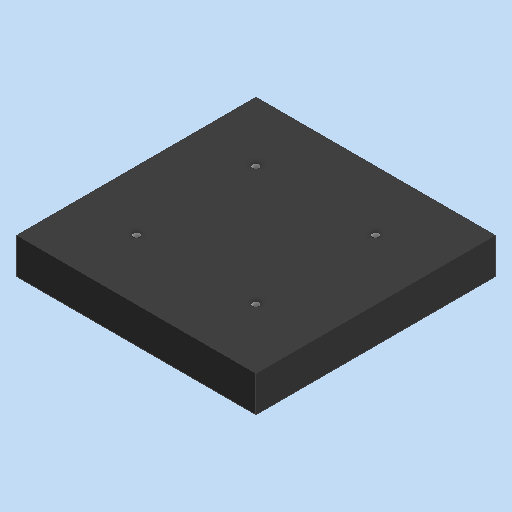
# Autodesk Inventor part: 底座
Saved by Autodesk Inventor 2026.2 (Build 302298010, 298A)
## iProperties
Created: 2026-03-16
Part Number: 底座
Material: 常规
Document SubType Name: Modeling
Designer: liu
Density: 1 g/cm^3
Appearance: 默认
Author: liu
Autodesk Inventor part; units mm, degrees
ref_plane "YZ Plane" through (0, 0, 0) normal (1, 0, 0) x (0, 1, 0)
ref_plane "XZ Plane" through (0, 0, 0) normal (0, 1, 0) x (-1, 0, 0)
ref_plane "XY Plane" through (0, 0, 0) normal (0, 0, 1) x (1, 0, 0)
sketch "草图1" plane through (0, 0, 0) normal (0, 1, 0) x (-1, 0, 0)
  line L0 (42.1224, 59.3469) -> (-57.8776, 59.3469)
  line L1 (-57.8776, 59.3469) -> (-57.8776, -40.6531)
  line L2 (-57.8776, -40.6531) -> (42.1224, -40.6531)
  line L3 (42.1224, -40.6531) -> (42.1224, 59.3469)
  point P0 (0, 0)
  dimension "d0" = 100
  dimension "d1" = 100
  constraints: 8 end point, 2 parallel, 1 horizontal, 1 perpendicular
  measures "d0" distance of L2.end L0.start
  measures "d1" distance of L1.end L2.end
extrude "拉伸1" add sketch "草图1" along normal blind 15
sketch "草图2" plane through (0, 15, 0) normal (0, 1, 0) x (1, 0, 0)
  circle A0 centre (-17.1224, -34.3469) radius 1.5
  line L0 (-42.1224, 40.6531) -> (-42.1224, -59.3469) projected
  line L1 (-42.1224, -59.3469) -> (57.8776, -59.3469) projected
  circle A1 centre (32.8776, -34.3469) radius 1.5
  circle A2 centre (32.8776, 15.6531) radius 1.5
  circle A3 centre (-17.1224, 15.6531) radius 1.5
  point P0 (0, 0)
  dimension "d4" = 3
  dimension "d5" = 25
  dimension "d6" = 25
  dimension "d9" = 50
  dimension "d16" = 50
  dimension "d23" = 50
  constraints: 4 centre point, 2 horizontal, 1 vertical, 6 other
  measures "d4" diameter of A0
  measures "d5" distance from line of L0 A0.centre
  measures "d6" distance from line of A0.centre L1
  measures "d9" distance of A0.centre A1.centre
  measures "d16" distance of A1.centre A2.centre
  measures "d23" distance of A2.centre A3.centre
extrude "拉伸2" cut sketch "草图2" against normal blind 15
